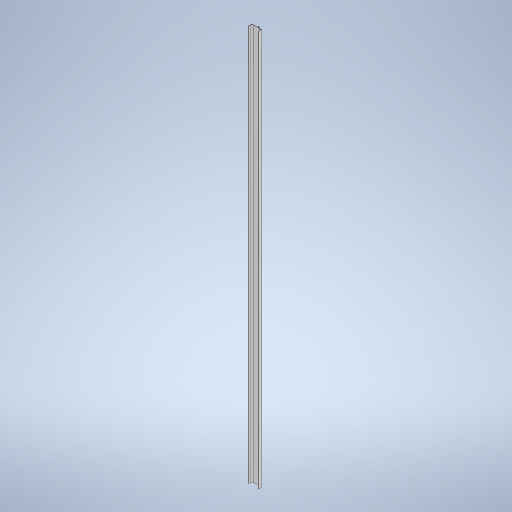
# Autodesk Inventor part: Hafele_alu_126_37_U-01
Saved by Autodesk Inventor 2024 (Build 280153000, 153)
## iProperties
RuleStatus: InUse
Created: 2019-10-04
Part Number: Hafele_alu_126_37_U-01
Material: Aluminum 6061
Document SubType Name: Modeling
Designer: RokasM
Density: 2.7 g/cm^3
Appearance: Aluminum - Polished
Author: RokasM
Autodesk Inventor part; units mm, degrees
ref_plane "YZ Plane" through (0, 0, 0) normal (1, 0, 0) x (0, 1, 0)
ref_plane "XZ Plane" through (0, 0, 0) normal (0, 1, 0) x (-1, 0, 0)
ref_plane "XY Plane" through (0, 0, 0) normal (0, 0, 1) x (1, 0, 0)
sketch "Sketch2" plane through (0, 0, 0) normal (0, 0, 1) x (1, 0, 0)
  line L0 (29.3, 0) -> (29.3, -22)
  line L1 (29.3, -22) -> (27.3, -22)
  line L2 (27.3, -22) -> (27.3, -12)
  arc A0 (27.3, -12) -> (17.3, -2) centre (17.3, -12) ccw
  line L3 (17.3, -2) -> (-20.7, -2)
  arc A1 (-20.7, -2) -> (-30.7, -12) centre (-20.7, -12) ccw
  line L4 (-30.7, -12) -> (-30.7, -22)
  line L5 (-30.7, -22) -> (-32.7, -22)
  line L6 (-32.7, -22) -> (-32.7, 0)
  line L7 (-32.7, 0) -> (-30.7, 0)
  line L8 (-30.7, 0) -> (-30.7, -5.3668)
  arc A2 (-20.7, 0) -> (-30.7, -5.3668) centre (-20.7, -12) ccw
  arc A3 (27.3, -5.3667) -> (17.3, 0) centre (17.3, -12) ccw
  line L9 (27.3, -5.3667) -> (27.3, 0)
  line L10 (27.3, 0) -> (29.3, 0)
  line L11 (2.15, 0) -> (2.15, 2)
  line L12 (2.15, 2) -> (1.65, 2)
  line L13 (1.65, 2) -> (2.15, 4)
  line L14 (2.15, 4) -> (1.65, 4)
  line L15 (1.65, 4) -> (2.15, 6)
  line L16 (2.15, 6) -> (1.65, 6)
  line L17 (1.65, 6) -> (2.15, 8)
  line L18 (2.15, 8) -> (1.65, 8)
  line L19 (1.65, 8) -> (2.15, 10)
  line L20 (2.15, 10) -> (3.85, 10)
  line L21 (3.85, 10) -> (4.35, 8)
  line L22 (4.35, 8) -> (3.85, 8)
  line L23 (3.85, 8) -> (4.35, 6)
  line L24 (4.35, 6) -> (3.85, 6)
  line L25 (3.85, 6) -> (4.35, 4)
  line L26 (4.35, 4) -> (3.85, 4)
  line L27 (3.85, 4) -> (4.35, 2)
  line L28 (4.35, 2) -> (3.85, 2)
  line L29 (3.85, 2) -> (3.85, 0)
  line L30 (17.3, 0) -> (3.85, 0)
  line L31 (2.15, 0) -> (-20.7, 0)
  point P0 (0, 0)
  point P1 (0, 0)
  dimension "d0" = 10
  dimension "d1" = 12
  dimension "d2" = 22
  dimension "d3" = 62
  dimension "d4" = 2
  dimension "d5" = 10
  dimension "d6" = 10
  dimension "d23" = 25.45
  dimension "d25" = 0.5
  dimension "d26" = 2
  dimension "d27" = 1.7
  dimension "d28" = 2
  dimension "d29" = 2.15
  dimension "d30" = 10
  dimension "d31" = 2
  dimension "d32" = 2
  dimension "d33" = 22
  dimension "d34" = 20
  dimension "d35" = 2
  dimension "d36" = 10
  dimension "d37" = 2
  dimension "d38" = 10
  constraints: 64 end point, 13 equal length, 10 parallel, 8 horizontal, 8 point on circle, 5 collinear, 4 centre point, 4 vertical alignment, 2 coincident, 2 concentric, 1 equal radius, 1 point on line
  measures "d0" radius of A1
  measures "d1" radius of A2
  measures "d2" distance between parallel lines of L1 L10
  measures "d3" distance between parallel lines of L6 L0
  measures "d4" distance between parallel lines of L8 L6
  measures "d5" distance from line of A1.centre L4
  measures "d6" distance from line of L3 A1.centre
  measures "d23" distance between parallel lines of L29 L0
  measures "d25" distance of L27.end L28.end
  measures "d26" distance between parallel lines of L24 L22
  measures "d27" distance between parallel lines of L11 L29
  measures "d28" distance from line of L3 point (0, 0)
  measures "d29" distance from line of point (0, 0) L11
  measures "d30" distance between parallel lines of L20 L30
  measures "d31" distance between parallel lines of L31 L3
  measures "d32" distance between parallel lines of L30 L3
  measures "d33" distance of L5.end L6.end
  measures "d34" distance between parallel lines of L3 L5
  measures "d35" distance of L9.end L0.start
  measures "d36" radius of A0
  measures "d37" distance between parallel lines of L0 L2
  measures "d38" distance from line of L3 A0.centre
extrude "01_ex1" add sketch "Sketch2" along normal blind 2500
fillet "Fillet2" radius 0.2 12 edges at (4.35, 8, 1250) (3.85, 10, 1250) (2.15, 10, 1250) (1.65, 8, 1250) (4.35, 6, 1250) (1.65, 6, 1250) (4.35, 4, 1250) (1.65, 4, 1250) (1.65, 2, 1250) (4.35, 2, 1250) (27.3, -5.3667, 1250) (-30.7, -5.3668, 1250)
fillet "Fillet2" radius 0.3 4 edges at (-30.7, -22, 1250) (-32.7, -22, 1250) (29.3, -22, 1250) (27.3, -22, 1250)
sketch "Sketch4" plane through (0, 0, 0) normal (0, 0, 1) x (1, 0, 0)
  line L0 (1.75, 11) -> (4.25, 11)
  line L1 (4.25, 11) -> (4.25, 0)
  line L2 (4.25, 0) -> (1.75, 0)
  line L3 (1.75, 0) -> (1.75, 11)
  line L4 (2.15, 0) -> (-20.7, 0) projected
  line L5 (3.85, 10) -> (2.15, 10) projected
  point P0 (0, 0)
  point P1 (3, 11)
  point P2 (3, 10)
  dimension "d41" = 2.5
  dimension "d42" = 11
  constraints: 8 end point, 2 midpoint, 2 parallel, 1 collinear, 1 horizontal, 1 perpendicular, 1 vertical alignment
  measures "d41" distance of L1.end L2.end
  measures "d42" distance of L0.end L1.end
extrude "02_ex1" add sketch "Sketch4" along normal blind 2500 separate body
ref_plane "Work Plane1" through (3, 2, 2500) normal (1, 0, 0) x (0, 0, -1)
equation "\"d5\" = d0"
equation "\"d6\" = d0"
equation "\"d39\" = Length"
equation "\"d43\" = Length"
equation "\"Length\" = 2500"
